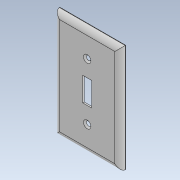
# Autodesk Inventor part: Light Switch Cover
Saved by Autodesk Inventor 2020.2 (Build 242310000, 310)
## iProperties
Created: 2020-04-30
Part Number: Light Switch Cover
Material: Generic
Document SubType Name: Modeling
Designer: Haashim Rehan
Density: 1 g/cm^3
Appearance: Default
Author: Haashim Rehan
Autodesk Inventor part; units mm, degrees
ref_plane "YZ Plane" through (0, 0, 0) normal (1, 0, 0) x (0, 1, 0)
ref_plane "XZ Plane" through (0, 0, 0) normal (0, 1, 0) x (-1, 0, 0)
ref_plane "XY Plane" through (0, 0, 0) normal (0, 0, 1) x (1, 0, 0)
sketch "Sketch1" plane through (0, 0, 0) normal (0, 0, 1) x (1, 0, 0)
  line L0 (-34.925, -57.15) -> (34.925, -57.15)
  line L1 (34.925, -57.15) -> (34.925, 57.15)
  line L2 (34.925, 57.15) -> (-34.925, 57.15)
  line L3 (-34.925, 57.15) -> (-34.925, -57.15)
  line L4 (-34.925, -57.15) -> (34.925, 57.15) construction
  line L5 (34.925, -57.15) -> (-34.925, 57.15) construction
  line L6 (-4.7625, -12.7) -> (4.7625, -12.7)
  line L7 (4.7625, -12.7) -> (4.7625, 12.7)
  line L8 (4.7625, 12.7) -> (-4.7625, 12.7)
  line L9 (-4.7625, 12.7) -> (-4.7625, -12.7)
  line L10 (-4.7625, -12.7) -> (4.7625, 12.7) construction
  line L11 (4.7625, -12.7) -> (-4.7625, 12.7) construction
  point P0 (0, 0)
  dimension "d0" = 69.85
  dimension "d1" = 114.3
  dimension "d2" = 9.525
  dimension "d3" = 25.4
  constraints: 24 end point, 4 midpoint, 4 parallel, 2 horizontal, 2 perpendicular
  measures "d0" distance of L2.end L1.end
  measures "d1" distance of L1.end L0.end
  measures "d2" distance of L8.end L7.end
  measures "d3" distance of L7.end L6.end
extrude "Extrusion1" add sketch "Sketch1" along normal blind 6
fillet "Fillet1" radius 5.5 4 edges at (0, 57.15, 6) (-34.925, 0, 6) (34.925, 0, 6) (0, -57.15, 6)
sketch "Sketch2" plane through (0, 0, 0) normal (0, 0, -1) x (-1, 0, 0)
  line L0 (-30.925, -53.15) -> (30.925, -53.15)
  line L1 (30.925, -53.15) -> (30.925, 53.15)
  line L2 (30.925, 53.15) -> (-30.925, 53.15)
  line L3 (-30.925, 53.15) -> (-30.925, -53.15)
  line L4 (-30.925, -53.15) -> (30.925, 53.15) construction
  line L5 (30.925, -53.15) -> (-30.925, 53.15) construction
  line L6 (-34.925, 57.15) -> (34.925, 57.15) projected
  line L7 (34.925, 57.15) -> (34.925, -57.15) projected
  point P0 (0, 0)
  dimension "d9" = 4
  dimension "d10" = 4
  constraints: 12 end point, 2 midpoint, 2 parallel, 1 horizontal, 1 perpendicular
  measures "d9" distance between parallel lines of L6 L2
  measures "d10" distance between parallel lines of L7 L1
extrude "Extrusion2" cut sketch "Sketch2" against normal blind 4.4
fillet "Fillet2" radius 2 8 edges at (-30.925, 0, 0) (0, -53.15, 0) (0, 53.15, 0) (0, 53.15, 4.4) (30.925, 0, 4.4) (-30.925, 0, 4.4) (30.925, 0, 0) (0, -53.15, 4.4)
sketch "Sketch3" plane through (0, 0, 6) normal (0, 0, 1) x (1, 0, 0)
  circle A0 centre (0, 30.15) radius 2.3813
  circle A1 centre (0, -30.15) radius 2.3813
  point P0 (0, 0)
  dimension "d14" = 60.3
  dimension "d15" = 4.7625
  dimension "d16" = 30.15
  dimension "d18" = 30.15
  constraints: 2 centre point, 2 vertical alignment, 1 equal radius
  measures "d14" distance of A1.centre A0.centre
  measures "d15" diameter of A0
  measures "d16" distance of point (0, 0) A0.centre
  measures "d18" distance of A1.centre point (0, 0)
extrude "Extrusion3" cut sketch "Sketch3" against normal through all
chamfer "Chamfer1" distance 1.6 angle 45 2 edges at (-2.3813, 30.15, 6) (-2.3813, -30.15, 6)
equation "\"d9\" = d10"
equation "\"d16\" = d18"
body "Solid1"
